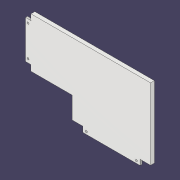
# Autodesk Inventor part: TC001b
Saved by Autodesk Inventor 2017 SP1 (Build 210196100, 196)
## iProperties
Created: 2018-01-07
Part Number: TC001b
Material: ABS Plastic
Document SubType Name: Modeling
Designer: Zach
Density: 1.06 g/cm^3
Appearance: CR White
Mass: 562.677 g
Surface Area: 1200.53 cm^2
Volume: 530.827 cm^3
Author: Zach
Autodesk Inventor part; units mm, degrees
ref_plane "YZ Plane" through (0, 0, 0) normal (1, 0, 0) x (0, 1, 0)
ref_plane "XZ Plane" through (0, 0, 0) normal (0, 1, 0) x (-1, 0, 0)
ref_plane "XY Plane" through (0, 0, 0) normal (0, 0, 1) x (1, 0, 0)
sketch "Sketch1" plane through (0, 0, 0) normal (0, 0, 1) x (1, 0, 0)
  line L0 (0, 0) -> (620, 0)
  line L1 (620, 0) -> (620, 620)
  line L2 (620, 620) -> (0, 620)
  line L3 (0, 620) -> (0, 0)
  line L4 (203, 491) -> (417, 491)
  line L5 (417, 491) -> (417, 377)
  line L6 (417, 377) -> (203, 377)
  line L7 (203, 377) -> (203, 491)
  point P0 (310, 491)
  point P1 (310, 620)
  dimension "d0" = 620
  dimension "d1" = 620
  dimension "d2" = 214
  dimension "d3" = 114
  dimension "d4" = 129
  constraints: 16 end point, 4 parallel, 2 horizontal, 2 midpoint, 2 perpendicular, 1 vertical alignment
  measures "d0" distance of L2.end L1.end
  measures "d1" distance of L1.end L0.end
  measures "d2" distance of L5.end L6.end
  measures "d3" distance of L4.end L5.end
  measures "d4" distance between parallel lines of L2 L4
extrude "Extrusion1" add sketch "Sketch1" along normal blind 10
sketch "Sketch2" plane through (0, 0, 10) normal (0, 0, 1) x (1, 0, 0)
  line L0 (0, 0) -> (310, 0)
  line L1 (310, 0) -> (310, 435)
  line L2 (310, 435) -> (0, 435)
  line L3 (0, 435) -> (0, 0)
  line L4 (620, 620) -> (0, 620) projected
  line L5 (0, 435) -> (620, 435)
  line L6 (620, 435) -> (620, 620)
  line L7 (620, 620) -> (0, 620)
  line L8 (0, 620) -> (0, 435)
  line L9 (310, 435) -> (620, 435)
  line L10 (620, 435) -> (620, 0)
  line L11 (620, 0) -> (310, 0)
  line L12 (310, 0) -> (310, 435)
  line L13 (0, 435) -> (310, 435)
  line L14 (310, 435) -> (310, 620)
  line L15 (310, 620) -> (0, 620)
  line L16 (0, 620) -> (0, 435)
  dimension "d7" = 435
  constraints: 32 end point, 8 parallel, 4 horizontal, 4 perpendicular, 1 midpoint, 1 vertical alignment
  measures "d7" distance of L1.end L0.end
extrude "Extrusion2" cut sketch "Sketch2" against normal through all contours L3 L2 L1 L0 | L1 L5 L10 L11 | L8 L4 L14 L2
sketch "Sketch6" plane through (0, 0, 10) normal (0, 0, 1) x (1, 0, 0)
  line L0 (310, 491) -> (310, 620) projected
  line L1 (310, 605) -> (296, 605)
  line L2 (296, 605) -> (296, 506)
  line L3 (296, 506) -> (310, 506)
  line L4 (310, 506) -> (310, 605)
  line L5 (417, 435) -> (620, 435) projected
  line L6 (444, 435) -> (593, 435)
  line L7 (593, 435) -> (593, 421)
  line L8 (593, 421) -> (444, 421)
  line L9 (444, 421) -> (444, 435)
  circle A0 centre (302.5, 595.5) radius 2.5
  circle A1 centre (302.5, 515.5) radius 2.5
  circle A2 centre (453.5, 427.5) radius 2.5
  circle A3 centre (583.5, 427.5) radius 2.5
  point P0 (0, 0)
  point P1 (310, 555.5)
  point P2 (518.5, 435)
  dimension "d28" = 14
  dimension "d29" = 99
  dimension "d30" = 149
  dimension "d31" = 14
  dimension "d32" = 5
  dimension "d33" = 5
  dimension "d34" = 9.5
  dimension "d35" = 9.5
  dimension "d36" = 7.5
  dimension "d37" = 7.5
  dimension "d38" = 5
  dimension "d39" = 5
  dimension "d40" = 9.5
  dimension "d41" = 9.5
  dimension "d42" = 7.5
  dimension "d43" = 7.5
  constraints: 16 end point, 4 centre point, 4 midpoint, 4 parallel, 2 horizontal, 2 perpendicular, 2 point on line
  measures "d28" distance of L3.end L2.end
  measures "d29" distance of L2.end L1.end
  measures "d30" distance of L7.end L8.end
  measures "d31" distance of L6.end L7.end
  measures "d32" diameter of A0
  measures "d33" diameter of A1
  measures "d34" distance from line of L1 A0.centre
  measures "d35" distance from line of L3 A1.centre
  measures "d36" distance from line of L4 A0.centre
  measures "d37" distance from line of L4 A1.centre
  measures "d38" diameter of A2
  measures "d39" diameter of A3
  measures "d40" distance from line of L7 A3.centre
  measures "d41" distance from line of L9 A2.centre
  measures "d42" distance from line of L5 A2.centre
  measures "d43" distance from line of L6 A3.centre
extrude "Extrusion6" add sketch "Sketch6" against normal blind 5
body "Solid1"
